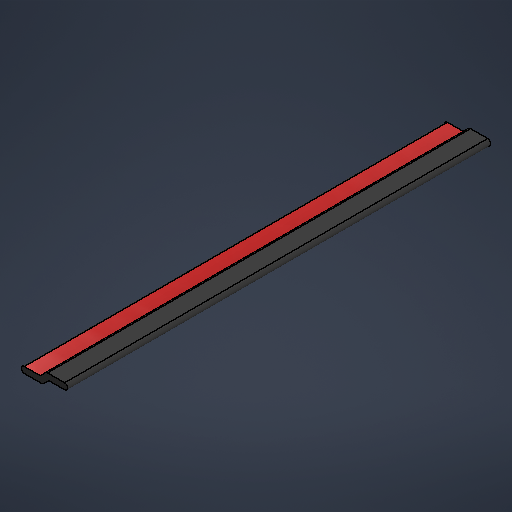
# Autodesk Inventor part: Door Seal
Saved by Autodesk Inventor 2026 (Build 300175050, 175E)
## iProperties
Created: 2025-05-22
Part Number: Door Seal
Material: Rubber
Document SubType Name: Modeling
Designer: Joshua Eah
Density: 0.93 g/cm^3
Appearance: Rubber - Black
Author: Joshua Eah
Autodesk Inventor part; units mm, degrees
ref_plane "YZ Plane" through (0, 0, 0) normal (1, 0, 0) x (0, 1, 0)
ref_plane "XZ Plane" through (0, 0, 0) normal (0, 1, 0) x (-1, 0, 0)
ref_plane "XY Plane" through (0, 0, 0) normal (0, 0, 1) x (1, 0, 0)
sketch "Sketch1" plane through (0, 0, 0) normal (0, 0, 1) x (1, 0, 0)
  line L0 (0, 0) -> (23, 0) construction
  line L1 (23, 0) -> (23, 6) construction
  line L2 (23, 6) -> (0, 6) construction
  line L3 (0, 6) -> (0, 0) construction
  line L4 (0, 3) -> (23, 3) construction
  line L5 (11.5, 0) -> (11.5, 3) construction
  line L6 (11.5, 3) -> (11.5, 6) construction
  line L7 (11.5, 1.5) -> (0, 1.5) construction
  line L8 (11.5, 4.5) -> (23, 4.5) construction
  line L9 (0, 1.5) -> (11.5, 1.5) construction
  line L10 (1.5, 3) -> (10, 3)
  line L11 (10, 0) -> (1.5, 0)
  arc A0 (1.5, 3) -> (1.5, 0) centre (1.5, 1.5) ccw
  arc A1 (10, 0) -> (10, 3) centre (10, 1.5) ccw
  line L12 (11.5, 4.5) -> (23, 4.5) construction
  line L13 (13, 6) -> (21.5, 6)
  line L14 (21.5, 3) -> (13, 3)
  arc A2 (13, 6) -> (13, 3) centre (13, 4.5) ccw
  arc A3 (21.5, 3) -> (21.5, 6) centre (21.5, 4.5) ccw
  line L15 (10, 1.5) -> (13, 4.5) construction
  line L16 (11.0607, 0.4393) -> (14.0607, 3.4393)
  line L17 (11.9393, 5.5607) -> (8.9393, 2.5607)
  arc A4 (8.9393, 2.5607) -> (11.0607, 0.4393) centre (10, 1.5) ccw
  arc A5 (14.0607, 3.4393) -> (11.9393, 5.5607) centre (13, 4.5) ccw
  point P0 (5.75, 1.5)
  point P1 (17.25, 4.5)
  point P2 (11.5, 3)
  point P3 (9.3787, 3)
  point P4 (13.6213, 3)
  dimension "d6" = 23
  dimension "d7" = 6
  dimension "d8" = 3
  constraints: 42 end point, 16 point on circle, 12 tangent, 10 midpoint, 7 equal length, 6 centre point, 6 point on line, 3 perpendicular, 2 concentric, 1 horizontal
  measures "d6" distance of L2.end L1.end
  measures "d7" distance of L1.end L0.end
  measures "d8" distance between parallel lines of L10 L11
extrude "Extrusion1" add sketch "Sketch1" along normal blind 210
body "Solid1"
